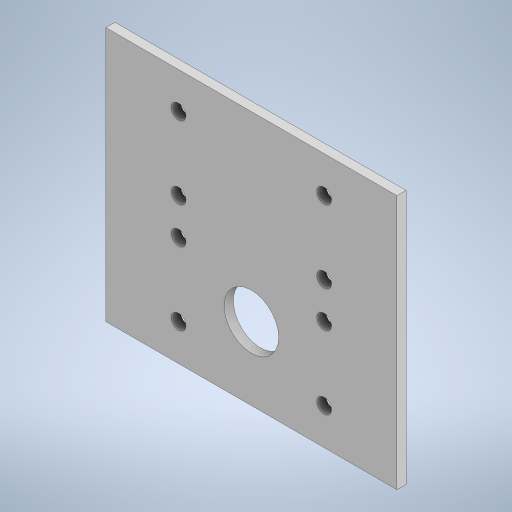
# Autodesk Inventor part: Dipper Plate
Saved by Autodesk Inventor 2023 (Build 270158000, 158)
## iProperties
Created: 2023-03-02
Part Number: Dipper Plate
Material: Generic
Document SubType Name: Modeling
Designer: Gabriel - T3 CAD
Density: 1 g/cm^3
Appearance: Default
Author: Gabriel - T3 CAD
Autodesk Inventor part; units mm, degrees
ref_plane "YZ Plane" through (0, 0, 0) normal (1, 0, 0) x (0, 1, 0)
ref_plane "XZ Plane" through (0, 0, 0) normal (0, 1, 0) x (-1, 0, 0)
ref_plane "XY Plane" through (0, 0, 0) normal (0, 0, 1) x (1, 0, 0)
sketch "Sketch1" plane through (0, 0, 0) normal (0, 0, 1) x (1, 0, 0)
  line L0 (0, 0) -> (-101.6, 0)
  line L1 (-101.6, 0) -> (-101.6, 88.9)
  line L2 (-101.6, 88.9) -> (0, 88.9)
  line L3 (0, 88.9) -> (0, 0)
  circle A0 centre (-76.2, 76.2) radius 2.5797
  circle A1 centre (-76.2, 50.8) radius 2.5797
  circle A2 centre (-25.4, 76.2) radius 2.5797
  circle A3 centre (-25.4, 50.8) radius 2.5797
  circle A4 centre (-50.8, 25.4) radius 9.525
  circle A5 centre (-76.2, 38.1) radius 2.5797
  circle A6 centre (-76.2, 12.7) radius 2.5797
  circle A7 centre (-25.4, 38.1) radius 2.5797
  circle A8 centre (-25.4, 12.7) radius 2.5797
  dimension "d0" = 101.6
  dimension "d1" = 88.9
  dimension "d4" = 25.4
  dimension "d7" = 50.8
  dimension "d10" = 12.7
  dimension "d11" = 25.4
  dimension "d12" = 5.1594
  dimension "d13" = 19.05
  dimension "d14" = 5.1594
  dimension "d17" = 25.4
  dimension "d20" = 50.8
  dimension "d23" = 25.4
  dimension "d24" = 12.7
  dimension "d25" = 25.4
  dimension "d26" = 50.8
  constraints: 9 centre point, 8 end point, 3 horizontal, 2 parallel, 2 vertical, 1 perpendicular, 12 other
  measures "d0" distance of L1.end L2.end
  measures "d1" distance of L0.end L1.end
  measures "d4" distance of A0.centre A1.centre
  measures "d7" distance of A0.centre A2.centre
  measures "d10" distance from line of L2 A0.centre
  measures "d11" distance from line of L1 A0.centre
  measures "d12" diameter of A0
  measures "d13" diameter of A4
  measures "d14" diameter of A5
  measures "d17" distance of A5.centre A6.centre
  measures "d20" distance of A5.centre A7.centre
  measures "d23" distance from line of L1 A5.centre
  measures "d24" distance from line of L0 A6.centre
  measures "d25" distance from line of L0 A4.centre
  measures "d26" distance from line of L1 A4.centre
extrude "Extrusion1" add sketch "Sketch1" along normal blind 3.175
body "Solid1"
